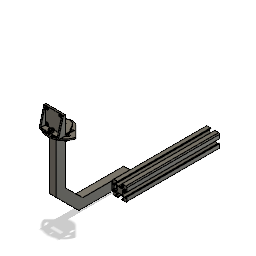
arducam_mk3_mount_v3 (Autodesk Fusion 360 design; units mm, degrees)
Autodesk Fusion 360 part; units mm, degrees
note: some values were not read from the file. Set by a fixed rule: which sketch regions a step uses.
sketch "Sketch1" plane through (0, 0, 0) normal (1, 0, 0) x (0, 0, -1)
sketch "Sketch2" plane through (0, 0, 0) normal (0, 0, 1) x (1, 0, 0)
  line L0 (8.8988, 5.095) -> (12.8205, 9.0167)
  line L1 (4, 0) -> (12.492, 0)
  line L2 (8.75, 2.765) -> (8.75, 4.7358)
  arc A0 (12.492, 0) -> (13, 0.508) centre (12.492, 0.508) ccw
  arc A1 (8.8988, 5.095) -> (8.75, 4.7358) centre (9.258, 4.7358) ccw
  line L3 (2, 10.492) -> (2, 2)
  line L4 (12.492, 2.257) -> (9.258, 2.257)
  arc A2 (2, 2) -> (4, 0) centre (4, 2) ccw
  arc A3 (13, 1.749) -> (12.492, 2.257) centre (12.492, 1.749) ccw
  line L5 (22.9833, 19.1808) -> (26.9037, 23.1012)
  arc A4 (13.1797, 9.1655) -> (12.8205, 9.0167) centre (13.1797, 8.6575) ccw
  arc A5 (27.2629, 23.25) -> (26.9037, 23.1012) centre (27.2629, 22.742) ccw
  arc A6 (21, 0.508) -> (21.508, 0) centre (21.508, 0.508) ccw
  line L6 (13, 0.508) -> (13, 1.749)
  arc A7 (8.75, 2.765) -> (9.258, 2.257) centre (9.258, 2.765) ccw
  line L7 (29.743, 10.492) -> (29.743, 7.258)
  line L8 (21, 1.749) -> (21, 0.508)
  arc A8 (22.8345, 11.1797) -> (22.9833, 10.8205) centre (23.3425, 11.1797) ccw
  line L9 (21.508, 0) -> (30, 0)
  arc A9 (25.25, 4.7371) -> (25.1012, 5.0963) centre (24.742, 4.7371) ccw
  arc A10 (24.742, 2.257) -> (25.25, 2.765) centre (24.742, 2.765) ccw
  arc A11 (22.9833, 19.1808) -> (22.8345, 18.8216) centre (23.3425, 18.8216) ccw
  arc A12 (30, 0) -> (32, 2) centre (30, 2) ccw
  line L10 (17.949, 9.1655) -> (20.8216, 9.1655)
  arc A13 (21.508, 2.257) -> (21, 1.749) centre (21.508, 1.749) ccw
  line L11 (26.905, 6.8988) -> (22.9833, 10.8205)
  arc A14 (21.1808, 9.0167) -> (20.8216, 9.1655) centre (20.8216, 8.6575) ccw
  line L12 (17, 9.675) -> (17.949, 9.1655)
  line L13 (22.8345, 11.1797) -> (22.8345, 14.051)
  line L14 (17.949, 20.8345) -> (17, 20.325)
  line L15 (32, 2) -> (32, 10.492)
  arc A15 (31.492, 19) -> (32, 19.508) centre (31.492, 19.508) ccw
  line L16 (22.8345, 15.949) -> (22.8345, 18.8216)
  line L17 (31.492, 11) -> (30.251, 11)
  line L18 (21.1808, 9.0167) -> (25.1012, 5.0963)
  arc A16 (25.25, 27.235) -> (24.742, 27.743) centre (24.742, 27.235) ccw
  arc A17 (12.8192, 20.9833) -> (13.1784, 20.8345) centre (13.1784, 21.3425) ccw
  arc A18 (20.8203, 20.8345) -> (21.1795, 20.9833) centre (20.8203, 21.3425) ccw
  arc A19 (30.251, 11) -> (29.743, 10.492) centre (30.251, 10.492) ccw
  arc A20 (32, 28) -> (30, 30) centre (30, 28) ccw
  arc A21 (8.75, 25.2629) -> (8.8988, 24.9037) centre (9.258, 25.2629) ccw
  line L19 (8.75, 25.2629) -> (8.75, 27.235)
  line L20 (25.25, 27.235) -> (25.25, 25.2642)
  arc A22 (25.1012, 24.905) -> (25.25, 25.2642) centre (24.742, 25.2642) ccw
  arc A23 (21.508, 30) -> (21, 29.492) centre (21.508, 29.492) ccw
  line L21 (22.325, 15) -> (22.8345, 15.949)
  line L22 (17, 20.325) -> (16.051, 20.8345)
  arc A24 (21, 28.251) -> (21.508, 27.743) centre (21.508, 28.251) ccw
  line L23 (22.8345, 14.051) -> (22.325, 15)
  line L24 (25.1012, 24.905) -> (21.1795, 20.9833)
  line L25 (13.1797, 9.1655) -> (16.051, 9.1655)
  arc A25 (32, 10.492) -> (31.492, 11) centre (31.492, 10.492) ccw
  line L26 (24.742, 2.257) -> (21.508, 2.257)
  line L27 (29.235, 6.75) -> (27.2642, 6.75)
  line L28 (25.25, 4.7371) -> (25.25, 2.765)
  arc A26 (26.905, 6.8988) -> (27.2642, 6.75) centre (27.2642, 7.258) ccw
  arc A27 (29.235, 6.75) -> (29.743, 7.258) centre (29.235, 7.258) ccw
  line L29 (16.051, 9.1655) -> (17, 9.675)
  arc A28 (12.492, 27.743) -> (13, 28.251) centre (12.492, 28.251) ccw
  line L30 (26.5, 5.119) -> (26.5, 1.681)
  arc A29 (30.7, 5.119) -> (30.319, 5.5) centre (30.319, 5.119) ccw
  line L31 (9.258, 27.743) -> (12.492, 27.743)
  line L32 (26.881, 1.3) -> (29.7, 1.3)
  line L33 (6.7371, 6.75) -> (4.765, 6.75)
  line L34 (30.251, 19) -> (31.492, 19)
  line L35 (21.508, 27.743) -> (24.742, 27.743)
  line L36 (29.743, 22.742) -> (29.743, 19.508)
  line L37 (32, 19.508) -> (32, 28)
  arc A30 (29.743, 19.508) -> (30.251, 19) centre (30.251, 19.508) ccw
  line L38 (12.492, 30) -> (4, 30)
  line L39 (20.8203, 20.8345) -> (17.949, 20.8345)
  line L40 (11.0167, 10.8192) -> (7.0963, 6.8988)
  line L41 (13, 28.251) -> (13, 29.492)
  line L42 (21, 29.492) -> (21, 28.251)
  arc A31 (4.765, 23.25) -> (4.257, 22.742) centre (4.765, 22.742) ccw
  line L43 (30.7, 2.3) -> (30.7, 5.119)
  arc A32 (11.0167, 10.8192) -> (11.1655, 11.1784) centre (10.6575, 11.1784) ccw
  arc A33 (26.881, 28.7) -> (26.5, 28.319) centre (26.881, 28.319) ccw
  arc A34 (29.743, 22.742) -> (29.235, 23.25) centre (29.235, 22.742) ccw
  line L44 (11.1655, 15.949) -> (11.675, 15)
  arc A35 (26.881, 5.5) -> (26.5, 5.119) centre (26.881, 5.119) ccw
  line L45 (11.675, 15) -> (11.1655, 14.051)
  arc A36 (13, 29.492) -> (12.492, 30) centre (12.492, 29.492) ccw
  arc A37 (4.257, 7.258) -> (4.765, 6.75) centre (4.765, 7.258) ccw
  arc A38 (4, 30) -> (2, 28) centre (4, 28) ccw
  line L46 (11.1655, 14.051) -> (11.1655, 11.1784)
  arc A39 (2, 19.508) -> (2.508, 19) centre (2.508, 19.508) ccw
  arc A40 (6.7371, 6.75) -> (7.0963, 6.8988) centre (6.7371, 7.258) ccw
  line L47 (4.765, 23.25) -> (6.7358, 23.25)
  line L48 (16.051, 20.8345) -> (13.1784, 20.8345)
  line L49 (11.1655, 18.8203) -> (11.1655, 15.949)
  line L50 (12.8192, 20.9833) -> (8.8988, 24.9037)
  line L51 (30, 30) -> (21.508, 30)
  line L52 (2, 28) -> (2, 19.508)
  arc A41 (9.258, 27.743) -> (8.75, 27.235) centre (9.258, 27.235) ccw
  line L53 (4.257, 19.508) -> (4.257, 22.742)
  line L54 (30.319, 5.5) -> (26.881, 5.5)
  line L55 (3.749, 11) -> (2.508, 11)
  arc A42 (7.095, 23.1012) -> (6.7358, 23.25) centre (6.7358, 22.742) ccw
  line L56 (2.508, 19) -> (3.749, 19)
  arc A43 (29.7, 1.3) -> (30.7, 2.3) centre (29.7, 2.3) ccw
  line L57 (4.257, 7.258) -> (4.257, 10.492)
  line L58 (7.095, 23.1012) -> (11.0167, 19.1795)
  line L59 (27.2629, 23.25) -> (29.235, 23.25)
  arc A44 (11.1655, 18.8203) -> (11.0167, 19.1795) centre (10.6575, 18.8203) ccw
  line L60 (26.5, 28.319) -> (26.5, 24.881)
  line L61 (4.3, 1.3) -> (7.119, 1.3)
  line L62 (13.8018, 13.5058) -> (12.9893, 12.4861)
  arc A45 (7.5, 28.319) -> (7.119, 28.7) centre (7.119, 28.319) ccw
  arc A46 (4.257, 10.492) -> (3.749, 11) centre (3.749, 10.492) ccw
  arc A47 (18.4942, 18.1982) -> (15.5058, 18.1982) centre (17, 15) ccw
  arc A48 (7.5, 5.119) -> (7.119, 5.5) centre (7.119, 5.119) ccw
  line L63 (15.5058, 18.1982) -> (14.4861, 19.0107)
  line L64 (14.4861, 10.9893) -> (15.5058, 11.8018)
  line L65 (7.119, 28.7) -> (4.3, 28.7)
  line L66 (7.5, 24.881) -> (7.5, 28.319)
  line L67 (30.7, 24.881) -> (30.7, 27.7)
  arc A49 (3.681, 5.5) -> (3.3, 5.119) centre (3.681, 5.119) ccw
  line L68 (18.4942, 11.8018) -> (19.5139, 10.9893)
  arc A50 (14.4861, 19.0107) -> (12.9893, 17.5139) centre (13.858, 18.142) ccw
  arc A51 (4.3, 28.7) -> (3.3, 27.7) centre (4.3, 27.7) ccw
  arc A52 (2.508, 11) -> (2, 10.492) centre (2.508, 10.492) ccw
  line L69 (12.9893, 17.5139) -> (13.8018, 16.4942)
  line L70 (21.0107, 12.4861) -> (20.1982, 13.5058)
  line L71 (3.681, 24.5) -> (7.119, 24.5)
  arc A53 (3.749, 19) -> (4.257, 19.508) centre (3.749, 19.508) ccw
  arc A54 (20.1982, 13.5058) -> (20.1982, 16.4942) centre (17, 15) ccw
  arc A55 (21.0107, 17.5139) -> (19.5139, 19.0107) centre (20.142, 18.142) ccw
  line L72 (7.119, 5.5) -> (3.681, 5.5)
  arc A56 (3.3, 2.3) -> (4.3, 1.3) centre (4.3, 2.3) ccw
  arc A57 (19.5139, 10.9893) -> (21.0107, 12.4861) centre (20.142, 11.858) ccw
  arc A58 (3.3, 24.881) -> (3.681, 24.5) centre (3.681, 24.881) ccw
  line L73 (29.7, 28.7) -> (26.881, 28.7)
  arc A59 (12.9893, 12.4861) -> (14.4861, 10.9893) centre (13.858, 11.858) ccw
  arc A60 (7.119, 1.3) -> (7.5, 1.681) centre (7.119, 1.681) ccw
  arc A61 (26.5, 24.881) -> (26.881, 24.5) centre (26.881, 24.881) ccw
  arc A62 (30.319, 24.5) -> (30.7, 24.881) centre (30.319, 24.881) ccw
  arc A63 (7.119, 24.5) -> (7.5, 24.881) centre (7.119, 24.881) ccw
  line L74 (3.3, 5.119) -> (3.3, 2.3)
  arc A64 (26.5, 1.681) -> (26.881, 1.3) centre (26.881, 1.681) ccw
  arc A65 (15.5058, 11.8018) -> (18.4942, 11.8018) centre (17, 15) ccw
  line L75 (3.3, 27.7) -> (3.3, 24.881)
  line L76 (7.5, 1.681) -> (7.5, 5.119)
  line L77 (20.1982, 16.4942) -> (21.0107, 17.5139)
  line L78 (19.5139, 19.0107) -> (18.4942, 18.1982)
  arc A66 (13.8018, 16.4942) -> (13.8018, 13.5058) centre (17, 15) ccw
  line L79 (26.881, 24.5) -> (30.319, 24.5)
  arc A67 (30.7, 27.7) -> (29.7, 28.7) centre (29.7, 27.7) ccw
extrude "Extrude1" add sketch "Sketch2" against normal blind 200 contours L0 L1 L2 A0 A1 L3 L4 A2 A3 L5 A4 A5 A6 L6 A7 L7 L8 A8 L9 A9 A10 A11 A12 L10 A13 L11 A14 L12 L13 L14 L15 A15 L16 L17 L18 A16 A17 A18 A19 A20 A21 L19 L20 A22 A23 L21 L22 A24 L23 L24 L25 A25 L26 L27 L28 A26 A27 L29 A28 L31 L33 L34 L35 L36 L37 A30 L38 L39 L40 L41 L42 A31 A32 A34 L44 L45 A36 A37 A38 L46 A39 A40 L47 L48 L49 L50 L51 L52 A41 L53 L55 A42 L56 L57 L58 L59 A44 A46 A52 A53 | L30 A29 L32 L43 A35 L54 A43 A64 | A33 L60 L67 L73 A61 A62 L79 A67 | L61 A48 A49 L72 A56 A60 L74 L76 | L62 A47 L63 L64 L68 A50 L69 L70 A54 A55 A57 A59 A65 L77 L78 A66 | A45 L65 L66 A51 L71 A58 A63 L75 makes body 1
ref_plane "WorkPlane1" through (0, 0, -40) normal (0, 0, 1) x (1, 0, 0)
sketch "Sketch3" plane through (0, 0, -40) normal (0, 0, 1) x (1, 0, 0)
  line L0 (0, 25) -> (-15, 25)
  line L1 (-15, 25) -> (-15, 5)
  line L2 (-15, 5) -> (0, 5)
  line L3 (0, 5) -> (0, 25)
  line L4 (2, 18.9) -> (4.5, 18.9)
  line L5 (4.5, 18.9) -> (4.5, 11.1)
  line L6 (4.5, 11.1) -> (2, 11.1)
  line L7 (2, 11.1) -> (2, 18.9)
  line L8 (0, 25) -> (2, 25)
  line L9 (2, 25) -> (2, 5)
  line L10 (2, 5) -> (0, 5)
  line L11 (0, 5) -> (0, 25)
  dimension "d6" = 15
  dimension "d7" = 20
  dimension "d8" = 5
  dimension "d9" = 7.8
  dimension "d10" = 2.5
  dimension "d11" = 6.1
  dimension "d280" = 2
  measures "d6" distance of L0.start L0.end
  measures "d7" distance of L0.start L2.end
  measures "d8" distance of origin L2
  measures "d9" distance of L4.end L5.end
  measures "d10" distance of L4.start L4.end
  measures "d11" distance of L2 L6
  measures "d280" distance of L0.start L8.end
extrude "Extrude2" add sketch "Sketch3" along normal blind 103 separate body contours L0 L1 L2 L3 L11 makes body 2
extrude "Extrude4" add sketch "Sketch3" along normal blind 40 contours L3 L7 L8 L9 L10 L11 | L4 L5 L6 L7 L9 bodies 2
sketch "Sketch5" plane through (-15, 0, 0) normal (-1, 0, 0) x (0, 0, 1)
  line L0 (-40, 25) -> (-40, 5)
  line L1 (-40, 5) -> (63, 5)
  line L2 (63, 5) -> (63, 25)
  line L3 (63, 25) -> (-40, 25)
  circle A0 centre (-30, 15) radius 2.6
  circle A1 centre (-10, 15) radius 2.6
  line L4 (0, 5) -> (0, 25) construction
  line L5 (-40, 15) -> (0, 15) construction
  dimension "d20" = 5.2
  dimension "d21" = 5.2
  dimension "d22" = 10
  dimension "d89" = 10
  measures "d20" diameter of A0
  measures "d21" diameter of A1
  measures "d22" distance of A0.centre L5.start
  measures "d89" distance of A1.centre L4
extrude "Extrude5" cut sketch "Sketch5" against normal through all contours A0 | A1 bodies 2
sketch "Sketch23" plane through (4.5, 0, 0) normal (1, 0, 0) x (0, 0, -1)
  circle A0 centre (30, 15) radius 2.6
  circle A1 centre (10, 15) radius 2.6
  line L0 (40, 11.1) -> (40, 18.9)
  line L1 (40, 18.9) -> (0, 18.9)
  line L2 (0, 18.9) -> (0, 11.1)
  line L3 (0, 11.1) -> (40, 11.1)
  line L4 (5.5, 18.9) -> (14.5, 18.9)
  line L5 (14.5, 18.9) -> (14.5, 11.1)
  line L6 (14.5, 11.1) -> (5.5, 11.1)
  line L7 (5.5, 11.1) -> (5.5, 18.9)
  line L8 (25.5, 18.9) -> (34.5, 18.9)
  line L9 (34.5, 18.9) -> (34.5, 11.1)
  line L10 (34.5, 11.1) -> (25.5, 11.1)
  line L11 (25.5, 11.1) -> (25.5, 18.9)
  dimension "d119" = 9
  dimension "d120" = 4.5
  dimension "d121" = 9
  dimension "d122" = 4.5
  measures "d119" distance of L9 L11
  measures "d120" distance of A0.centre L11
  measures "d121" distance of L5 L7
  measures "d122" distance of A1.centre L7
extrude "Extrude19" cut sketch "Sketch23" against normal blind 2.5 contours L1 L3 L8 L9 L10 L11 | L1 L3 L4 L5 L6 L7 bodies 2
sketch "Sketch6" plane through (-15, 0, 0) normal (-1, 0, 0) x (0, 0, 1)
  line L0 (63, 5) -> (120, 62) construction
  line L1 (63, 5) -> (136.0301, 5) construction
  line L2 (120, 62) -> (100, 62) construction
  line L3 (100, 62) -> (63, 25)
  line L4 (100, 62) -> (100, 172)
  line L5 (120, 62) -> (120, 172)
  line L6 (120, 172) -> (100, 172) construction
  line L7 (63, 25) -> (63, 5)
  line L8 (63, 5) -> (71.2843, 5)
  line L9 (71.2843, 5) -> (120, 53.7157)
  line L10 (120, 62) -> (120, 53.7157)
  arc A0 (120, 172) -> (100, 172) centre (110, 172) ccw
  circle A1 centre (110, 172) radius 2.6
  point P0 (63, 5)
  point P1 (63, 25)
  dimension "d32" = 45
  dimension "d35" = 37
  dimension "d36" = 110
  dimension "d145" = 20
  dimension "d146" = 5.2
  measures "d32" angle of L0 L1
  measures "d35" distance of L2.end P1
  measures "d36" distance of L2.end L4.end
  measures "d145" distance of L3 L9
  measures "d146" diameter of A1
extrude "Extrude6" add sketch "Sketch6" against normal blind 15 bodies 2
sketch "Sketch28" plane through (0, 0, 0) normal (1, 0, 0) x (0, 0, -1)
  line L0 (5.5, 11.1) -> (0, 11.1)
  line L1 (0, 11.1) -> (0, 5)
  line L2 (0, 18.9) -> (5.5, 18.9)
  line L3 (5.5, 18.9) -> (5.5, 11.1)
  circle A0 centre (10, 15) radius 2.6
  line L4 (14.5, 11.1) -> (14.5, 18.9)
  line L5 (14.5, 18.9) -> (25.5, 18.9)
  line L6 (25.5, 18.9) -> (25.5, 11.1)
  line L7 (25.5, 11.1) -> (14.5, 11.1)
  circle A1 centre (30, 15) radius 2.6
  line L8 (34.5, 11.1) -> (34.5, 18.9)
  line L9 (34.5, 18.9) -> (40, 18.9)
  line L10 (40, 18.9) -> (40, 25)
  line L11 (40, 25) -> (0, 25)
  line L12 (0, 5) -> (40, 5)
  line L13 (40, 5) -> (40, 11.1)
  line L14 (40, 11.1) -> (34.5, 11.1)
  arc A2 (-120, 172) -> (-100, 172) centre (-110, 172) ccw
  line L15 (-120, 172) -> (-120, 184)
  line L16 (-120, 184) -> (-117, 184)
  line L17 (-117, 184) -> (-117, 187)
  line L18 (-117, 187) -> (-103, 187)
  line L19 (-103, 187) -> (-103, 184)
  line L20 (-103, 184) -> (-100, 184)
  line L21 (-100, 184) -> (-100, 172)
  line L22 (0, 25) -> (0, 18.9)
  dimension "d187" = 15
  dimension "d188" = 3
  dimension "d189" = 3
  measures "d187" distance of A2.centre L18
  measures "d188" distance of L16 L18
  measures "d189" distance of L15 L17
extrude "Extrude31" add sketch "Sketch28" along normal blind 15 separate body contours A2 L15 L16 L17 L18 L19 L20 L21 makes body 3
sketch "Sketch38" plane through (15, 0, 0) normal (1, 0, 0) x (0, 0, -1)
  arc A0 (-120, 172) -> (-100, 172) centre (-110, 172) ccw
  line L0 (-100, 172) -> (-100, 184)
  line L1 (-100, 184) -> (-103, 184)
  line L2 (-103, 184) -> (-103, 187)
  line L3 (-103, 187) -> (-117, 187)
  line L4 (-117, 187) -> (-117, 184)
  line L5 (-117, 184) -> (-120, 184)
  line L6 (-120, 184) -> (-120, 172)
  line L7 (-112.3671, 176.1) -> (-114.7343, 172)
  line L8 (-114.7343, 172) -> (-112.3671, 167.9)
  line L9 (-112.3671, 167.9) -> (-107.6329, 167.9)
  line L10 (-107.6329, 167.9) -> (-105.2657, 172)
  line L11 (-105.2657, 172) -> (-107.6329, 176.1)
  line L12 (-107.6329, 176.1) -> (-112.3671, 176.1)
  point P0 (-110, 172)
  dimension "d192" = 4.1
  measures "d192" distance of P0 L12
extrude "Extrude32" cut sketch "Sketch38" against normal blind 5 contours L7 L8 L9 L10 L11 L12 bodies 3
sketch "Sketch39" plane through (0, 187, 0) normal (0, 1, 0) x (-1, 0, 0)
  line L0 (0, 103) -> (0, 117)
  line L1 (0, 117) -> (-15, 117)
  line L2 (-15, 117) -> (-15, 103)
  line L3 (-15, 103) -> (0, 103)
  line L4 (0, 103) -> (-15, 117) construction
  line L5 (0, 117) -> (-15, 103) construction
  circle A0 centre (-7.5, 110) radius 2.5
  dimension "d195" = 5
  measures "d195" diameter of A0
extrude "Extrude33" cut sketch "Sketch39" against normal blind 6 contours A0 bodies 3
ref_plane "WorkPlane10" through (7.5, 187.2, 110) normal (0, 1, 0) x (0, 0, 1)
sketch "Sketch40" plane through (7.5, 187.2, 110) normal (0, 1, 0) x (1, 0, 0)
  circle A0 centre (0, 0) radius 2.5 construction
  circle A1 centre (0, 0) radius 2.65
  line L0 (-18, -19) -> (18, -19) construction
  line L1 (18, -19) -> (18, -23) construction
  line L2 (18, -23) -> (-18, -23) construction
  line L3 (-18, -23) -> (-18, -19) construction
  line L4 (-10.5973, 6.6293) -> (-21, -10)
  line L5 (-21, -10) -> (-21, -33)
  line L6 (-21, -33) -> (21, -33)
  line L7 (21, -33) -> (21, -10)
  line L8 (21, -10) -> (10.5973, 6.6293)
  line L9 (-18, -19) -> (-18, -13) construction
  line L10 (-18, -13) -> (18, -13) construction
  line L11 (18, -19) -> (18, -13) construction
  line L12 (-21, -10) -> (21, -10) construction
  arc A2 (10.5973, 6.6293) -> (-10.5973, 6.6293) centre (0, 0) ccw
  dimension "d199" = 5.3
  dimension "d200" = 25
  dimension "d202" = 36
  dimension "d203" = 18
  dimension "d204" = 19
  dimension "d205" = 4
  dimension "d207" = 3
  dimension "d208" = 3
  dimension "d209" = 10
  dimension "d210" = 6
  dimension "d211" = 3
  measures "d199" diameter of A1
  measures "d200" diameter of A2
  measures "d202" distance of L1 L3
  measures "d203" distance of A0.centre L1
  measures "d204" distance of A0.centre L0
  measures "d205" distance of L0 L2
  measures "d207" distance of L1 L7
  measures "d208" distance of L3 L5
  measures "d209" distance of L2 L6
  measures "d210" distance of L0 L10
  measures "d211" distance of L4.end L10
extrude "Extrude34" add sketch "Sketch40" along normal blind 3 separate body makes body 4
sketch "Sketch41" plane through (0, 190.2, 0) normal (0, 1, 0) x (-1, 0, 0)
  circle A0 centre (-7.5, 110) radius 2.65
  arc A1 (-18.0973, 103.3707) -> (3.0973, 103.3707) centre (-7.5, 110) ccw
  line L0 (3.0973, 103.3707) -> (13.5, 120)
  line L1 (13.5, 120) -> (13.5, 143)
  line L2 (13.5, 143) -> (-28.5, 143)
  line L3 (-28.5, 143) -> (-28.5, 120)
  line L4 (-28.5, 120) -> (-18.0973, 103.3707)
  line L5 (13.5, 129) -> (-28.5, 129)
  line L6 (-28.5, 129) -> (-28.5, 133)
  line L7 (-28.5, 133) -> (13.5, 133)
  line L8 (13.5, 133) -> (13.5, 129)
  dimension "d214" = 4
  dimension "d215" = 10
  measures "d214" distance of L5 L7
  measures "d215" distance of L2 L7
extrude "Extrude35" add sketch "Sketch41" along normal blind 37 contours L1 L3 L5 L6 L7 L8 bodies 4
sketch "Sketch42" plane through (28.5, 0, 0) normal (1, 0, 0) x (0, 0, -1)
  line L0 (-143, 187.2) -> (-120, 187.2)
  line L1 (-120, 187.2) -> (-120, 190.2)
  line L2 (-120, 190.2) -> (-129, 190.2)
  line L3 (-129, 190.2) -> (-129, 227.2)
  line L4 (-129, 227.2) -> (-133, 227.2)
  line L5 (-133, 227.2) -> (-133, 190.2)
  line L6 (-133, 190.2) -> (-143, 190.2)
  line L7 (-143, 190.2) -> (-143, 187.2)
  line L8 (-133, 227.2) -> (-143, 190.2)
  line L9 (-133, 227.2) -> (-133, 190.2)
  line L10 (-143, 190.2) -> (-133, 190.2)
extrude "Extrude36" add sketch "Sketch42" against normal blind 3 contours L5 L6 L8 L9 L10 bodies 4
sketch "Sketch43" plane through (-13.5, 0, 0) normal (-1, 0, 0) x (0, 0, 1)
  line L0 (120, 187.2) -> (143, 187.2)
  line L1 (143, 187.2) -> (143, 190.2)
  line L2 (143, 190.2) -> (133, 190.2)
  line L3 (133, 190.2) -> (133, 227.2)
  line L4 (133, 227.2) -> (129, 227.2)
  line L5 (129, 227.2) -> (129, 190.2)
  line L6 (129, 190.2) -> (120, 190.2)
  line L7 (120, 190.2) -> (120, 187.2)
  line L8 (133, 227.2) -> (143, 190.2)
  line L9 (143, 190.2) -> (133, 190.2)
  line L10 (133, 227.2) -> (133, 190.2)
extrude "Extrude37" add sketch "Sketch43" against normal blind 3 contours L2 L3 L8 L9 L10 bodies 4
sketch "Sketch44" plane through (0, 0, 129) normal (0, 0, -1) x (-1, 0, 0)
  line L0 (-28.5, 190.2) -> (13.5, 190.2)
  line L1 (13.5, 190.2) -> (13.5, 227.2)
  line L2 (13.5, 227.2) -> (-28.5, 227.2)
  line L3 (-28.5, 227.2) -> (-28.5, 190.2)
  line L4 (-25.5, 226.7) -> (10.5, 226.7) construction
  line L5 (10.5, 226.7) -> (10.5, 190.7) construction
  line L6 (10.5, 190.7) -> (-25.5, 190.7) construction
  line L7 (-25.5, 190.7) -> (-25.5, 226.7) construction
  line L8 (-28.5, 208.7) -> (13.5, 208.7) construction
  line L9 (-7.5, 227.2) -> (-7.5, 190.2) construction
  circle A0 centre (-21.9, 223.1) radius 1.6
  circle A1 centre (6.9, 223.1) radius 1.6
  circle A2 centre (-21.9, 194.3) radius 1.6
  circle A3 centre (6.9, 194.3) radius 1.6
  dimension "d222" = 36
  dimension "d223" = 36
  dimension "d224" = 18
  dimension "d225" = 18
  dimension "d226" = 3.2
  dimension "d227" = 14.4
  dimension "d228" = 14.4
  measures "d222" distance of L4.start L4.end
  measures "d223" distance of L4.end L5.end
  measures "d224" distance of L4 L8
  measures "d225" distance of L7 L9
  measures "d226" diameter of A0
  measures "d227" distance of L9 A0.centre
  measures "d228" distance of L8 A0.centre
extrude "Extrude38" cut sketch "Sketch44" against normal through all contours A0 | A1 | A2 | A3 bodies 4
sketch "Sketch45" plane through (0, 0, 133) normal (0, 0, 1) x (1, 0, 0)
  circle A0 centre (-6.9, 223.1) radius 1.6
  circle A1 centre (-6.9, 194.3) radius 1.6
  circle A2 centre (21.9, 223.1) radius 1.6
  circle A3 centre (21.9, 194.3) radius 1.6
  line L0 (-10.5, 227.2) -> (-10.5, 190.2)
  line L1 (-10.5, 190.2) -> (25.5, 190.2)
  line L2 (25.5, 190.2) -> (25.5, 227.2)
  line L3 (25.5, 227.2) -> (-10.5, 227.2)
  circle A4 centre (-6.9, 223.1) radius 1.6 construction
  circle A5 centre (21.9, 223.1) radius 1.6 construction
  circle A6 centre (21.9, 194.3) radius 1.6 construction
  circle A7 centre (-6.9, 194.3) radius 1.6 construction
  line L4 (-4.05, 224.7454) -> (-6.9, 226.3909)
  line L5 (-6.9, 226.3909) -> (-9.75, 224.7454)
  line L6 (-9.75, 224.7454) -> (-9.75, 221.4546)
  line L7 (-9.75, 221.4546) -> (-6.9, 219.8091)
  line L8 (-6.9, 219.8091) -> (-4.05, 221.4546)
  line L9 (-4.05, 221.4546) -> (-4.05, 224.7454)
  line L10 (19.05, 221.4546) -> (21.9, 219.8091)
  line L11 (21.9, 219.8091) -> (24.75, 221.4546)
  line L12 (24.75, 221.4546) -> (24.75, 224.7454)
  line L13 (24.75, 224.7454) -> (21.9, 226.3909)
  line L14 (21.9, 226.3909) -> (19.05, 224.7454)
  line L15 (19.05, 224.7454) -> (19.05, 221.4546)
  line L16 (-4.05, 195.9454) -> (-6.9, 197.5909)
  line L17 (-6.9, 197.5909) -> (-9.75, 195.9454)
  line L18 (-9.75, 195.9454) -> (-9.75, 192.6546)
  line L19 (-9.75, 192.6546) -> (-6.9, 191.0091)
  line L20 (-6.9, 191.0091) -> (-4.05, 192.6546)
  line L21 (-4.05, 192.6546) -> (-4.05, 195.9454)
  line L22 (19.05, 192.6546) -> (21.9, 191.0091)
  line L23 (21.9, 191.0091) -> (24.75, 192.6546)
  line L24 (24.75, 192.6546) -> (24.75, 195.9454)
  line L25 (24.75, 195.9454) -> (21.9, 197.5909)
  line L26 (21.9, 197.5909) -> (19.05, 195.9454)
  line L27 (19.05, 195.9454) -> (19.05, 192.6546)
  point P0 (-6.9, 223.1)
  point P1 (21.9, 223.1)
  point P2 (-6.9, 194.3)
  point P3 (21.9, 194.3)
  dimension "d230" = 2.85
  dimension "d231" = 2.85
  dimension "d232" = 2.85
  dimension "d233" = 2.85
  measures "d230" distance of P0 L9
  measures "d231" distance of P1 L15
  measures "d232" distance of P2 L21
  measures "d233" distance of P3 L27
extrude "Extrude39" cut sketch "Sketch45" against normal blind 1 contours L4 L5 L6 L7 L8 L9 | L10 L11 L12 L13 L14 L15 | L16 L17 L18 L19 L20 L21 | L22 L23 L24 L25 L26 L27 bodies 4
sketch "Sketch46" plane through (0, 190.2, 0) normal (0, 1, 0) x (-1, 0, 0)
  line L0 (13.5, 129) -> (-28.5, 129)
  line L1 (-28.5, 129) -> (-28.5, 120)
  line L2 (-28.5, 120) -> (-18.0973, 103.3707)
  arc A0 (-18.0973, 103.3707) -> (3.0973, 103.3707) centre (-7.5, 110) ccw
  line L3 (3.0973, 103.3707) -> (13.5, 120)
  line L4 (13.5, 120) -> (13.5, 129)
  circle A1 centre (-7.5, 110) radius 2.65
  line L5 (-18.5, 127.4) -> (3.5, 127.4)
  line L6 (3.5, 127.4) -> (3.5, 124.9)
  line L7 (3.5, 124.9) -> (-18.5, 124.9)
  line L8 (-18.5, 124.9) -> (-18.5, 127.4)
  circle A2 centre (-7.5, 110) radius 2.65 construction
  dimension "d236" = 2.5
  dimension "d237" = 1.6
  dimension "d238" = 22
  dimension "d239" = 11
  measures "d236" distance of L5.start L7.end
  measures "d237" distance of L0 L5
  measures "d238" distance of L6 L8
  measures "d239" distance of L6 A0.centre
extrude "Extrude40" cut sketch "Sketch46" against normal through all contours L5 L6 L7 L8 bodies 4
sketch "Sketch47" plane through (0, 190.2, 0) normal (0, 1, 0) x (-1, 0, 0)
  line L0 (10.5, 133) -> (10.5, 143)
  line L1 (10.5, 143) -> (-25.5, 143)
  line L2 (-25.5, 143) -> (-25.5, 133)
  line L3 (-25.5, 133) -> (10.5, 133)
  line L4 (-7.5, 133) -> (-7.5, 143) construction
  line L5 (10.5, 138) -> (-25.5, 138) construction
  circle A0 centre (-7.5, 138) radius 1.55
  line L6 (-9.1454, 140.85) -> (-10.7909, 138)
  line L7 (-10.7909, 138) -> (-9.1454, 135.15)
  line L8 (-9.1454, 135.15) -> (-5.8546, 135.15)
  line L9 (-5.8546, 135.15) -> (-4.2091, 138)
  line L10 (-4.2091, 138) -> (-5.8546, 140.85)
  line L11 (-5.8546, 140.85) -> (-9.1454, 140.85)
  line L12 (-10.0115, 142.35) -> (-12.5229, 138)
  line L13 (-12.5229, 138) -> (-10.0115, 133.65)
  line L14 (-10.0115, 133.65) -> (-4.9885, 133.65)
  line L15 (-4.9885, 133.65) -> (-2.4771, 138)
  line L16 (-2.4771, 138) -> (-4.9885, 142.35)
  line L17 (-4.9885, 142.35) -> (-10.0115, 142.35)
  point P0 (-7.5, 138)
  dimension "d241" = 3.1
  dimension "d242" = 2.85
  dimension "d243" = 1.5
  measures "d241" diameter of A0
  measures "d242" distance of P0 L11
extrude "Extrude41" add sketch "Sketch47" along normal blind 3 contours L12 L13 L14 L15 L16 L17 bodies 4
extrude "Extrude42" cut sketch "Sketch47" against normal through all contours A0 bodies 4
sketch "Sketch48" plane through (0, 184, 0) normal (0, 1, 0) x (-1, 0, 0)
  line L0 (0, 117) -> (0, 120)
  line L1 (0, 120) -> (-15, 120)
  line L2 (-15, 120) -> (-15, 117)
  line L3 (-15, 117) -> (0, 117)
  circle A0 centre (-7.5, 110) radius 2.65 construction
  circle A1 centre (-7.5, 138) radius 1.55 construction
  circle A2 centre (-7.5, 110) radius 26.45 construction
  circle A3 centre (-7.5, 110) radius 29.55 construction
  line L4 (-7.5, 110) -> (18.0911, 124.775) construction
  line L5 (-7.5, 110) -> (22.05, 110) construction
  line L6 (-7.5, 110) -> (-33.0911, 124.775) construction
  circle A4 centre (-7.5, 110) radius 28 construction
  circle A5 centre (16.7487, 124) radius 1.55 construction
  circle A6 centre (-31.7487, 124) radius 1.55 construction
  arc A7 (-33.3509, 124.925) -> (-30.1466, 123.075) centre (-31.7487, 124) ccw
  arc A8 (15.1466, 123.075) -> (18.3509, 124.925) centre (16.7487, 124) ccw
  arc A9 (18.3509, 124.925) -> (-33.3509, 124.925) centre (-7.5, 110) ccw
  arc A10 (15.1466, 123.075) -> (-30.1466, 123.075) centre (-7.5, 110) ccw
  dimension "d247" = 30
  dimension "d248" = 150
  dimension "d253" = 26.15
  dimension "d254" = 29.85
  measures "d247" angle of L4 L5
  measures "d248" angle of L5 L6
  measures "d253" radius of A10
  measures "d254" radius of A9
sketch "Sketch49" plane through (0, 184, 0) normal (0, 1, 0) x (-1, 0, 0)
  line L0 (-15, 117) -> (0, 117)
  line L1 (0, 103) -> (-15, 103) construction
  line L2 (0, 117) -> (0, 103) construction
  line L3 (0, 117) -> (-15, 117) construction
  line L4 (-15, 103) -> (-15, 117) construction
  line L5 (0.1, 102.9) -> (-15.1, 102.9)
  line L6 (-15.1, 102.9) -> (-15.1, 117.1)
  line L7 (-15.1, 117.1) -> (0.1, 117.1)
  line L8 (0.1, 117.1) -> (0.1, 102.9)
  arc A0 (27.1823, 119.6507) -> (-42.1823, 119.6507) centre (-7.5, 110) ccw
  arc A1 (-20.0158, 97.4842) -> (5.0158, 97.4842) centre (-7.5, 110) ccw
  line L9 (27.1823, 119.6507) -> (5.0158, 97.4842)
  line L10 (-20.0158, 97.4842) -> (-42.1823, 119.6507)
  line L11 (-7.5, 110) -> (-7.5, 146.007) construction
  point P0 (-7.5, 110)
  dimension "d255" = 0.1
  dimension "d256" = 0.1
  dimension "d257" = 0.1
  dimension "d258" = 0.1
  dimension "d267" = 36
  dimension "d276" = 17.7
  dimension "d277" = 45
  dimension "d278" = 45
  measures "d255" distance of L1 L5
  measures "d256" distance of L0 L7
  measures "d257" distance of L4 L6
  measures "d258" distance of L2 L8
  measures "d267" radius of A0
  measures "d276" radius of A1
  measures "d277" angle of L9 L11
  measures "d278" angle of L10 L11
extrude "Extrude43" add sketch "Sketch49" along normal blind 3 separate body makes body 5
extrude "Extrude44" cut sketch "Sketch48" along normal through all contours A7 A8 A9 A10 bodies 5
sketch "Sketch50" plane through (0, 184, 0) normal (0, 1, 0) x (-1, 0, 0)
  line L0 (-18.5, 124.9) -> (-18.5, 127.4) construction
  line L1 (-18.5, 127.4) -> (3.5, 127.4) construction
  line L2 (3.5, 127.4) -> (3.5, 124.9) construction
  line L3 (3.5, 124.9) -> (-18.5, 124.9) construction
  circle A0 centre (-7.5, 110) radius 2.65 construction
  line L4 (-18.5, 124.9) -> (-18.5, 127.4) construction
  line L5 (-18.5, 127.4) -> (3.5, 127.4) construction
  line L6 (3.5, 127.4) -> (3.5, 124.9) construction
  circle A1 centre (-7.5, 110) radius 2.65 construction
  line L7 (3.5, 124.9) -> (-18.5, 124.9) construction
  line L8 (-18.5, 124.9) -> (-18.5, 127.4) construction
  line L9 (-18.5, 127.4) -> (3.5, 127.4) construction
  line L10 (3.5, 127.4) -> (3.5, 124.9) construction
  line L11 (-14.9038, 126.9763) -> (-25.9038, 107.9237) construction
  line L12 (-28.0688, 109.1737) -> (-17.0688, 128.2263) construction
  line L13 (-25.9038, 107.9237) -> (-28.0688, 109.1737) construction
  line L14 (-17.0688, 128.2263) -> (-14.9038, 126.9763) construction
  circle A2 centre (-7.5, 110) radius 20.5854 construction
  line L15 (-7.5, 110) -> (-7.5, 130.5854) construction
  line L16 (-0.0962, 126.9763) -> (10.9038, 107.9237) construction
  line L17 (10.9038, 107.9237) -> (13.0688, 109.1737) construction
  line L18 (13.0688, 109.1737) -> (2.0688, 128.2263) construction
  line L19 (2.0688, 128.2263) -> (-0.0962, 126.9763) construction
  line L20 (13.0688, 109.1737) -> (10.9038, 107.9237)
  line L21 (5.4038, 117.45) -> (10.9038, 107.9237)
  line L22 (-20.4038, 117.45) -> (-25.9038, 107.9237)
  line L23 (-25.9038, 107.9237) -> (-28.0688, 109.1737)
  arc A3 (13.0688, 109.1737) -> (-28.0688, 109.1737) centre (-7.5, 110) ccw
  arc A4 (5.4038, 117.45) -> (-20.4038, 117.45) centre (-7.5, 110) ccw construction
  arc A5 (5.4038, 117.45) -> (-20.4038, 117.45) centre (-7.5, 110) ccw
  point P0 (-18.5284, 124.8763)
extrude "Extrude45" cut sketch "Sketch50" along normal blind 3 bodies 5
equation "d8 = ( 30 mm - d7 ) / 2"
equation "d11 = ( d7 - d9 ) / 2"
equation "d21 = d20"
equation "d89 = d22"
equation "d120 = d119 / 2"
equation "d121 = d119"
equation "d122 = d121 / 2"
equation "d203 = d202 / 2"
equation "d224 = d223 / 2"
equation "d225 = d222 / 2"
equation "d227 = ( 28.8 / 2 ) * 1 mm"
equation "d228 = ( 28.8 / 2 ) * 1 mm"
equation "d231 = d230"
equation "d232 = d230"
equation "d233 = d230"
equation "d239 = d238 / 2"
equation "d242 = ( ( 5.5 / 2 ) + 0.1 ) * 1 mm"
equation "d256 = d255"
equation "d257 = d255"
equation "d258 = d255"
equation "d278 = d277"
named bodies: "rail_sample", "rail_arm", "pivot_arm", "rotation_body", "rotation_plate"
